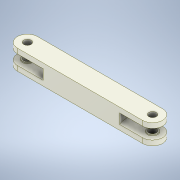
# Autodesk Inventor part: LinkB
Saved by Autodesk Inventor 2022 (Build 260153000, 153)
## iProperties
Created: 2021-11-22
Part Number: LinkB
Material: Plástico ABS
Document SubType Name: Modeling
Designer: JK
Density: 1.06 g/cm^3
Appearance: Suave - Marfil
Author: JK
Autodesk Inventor part; units mm, degrees
ref_plane "YZ Plane" through (0, 0, 0) normal (1, 0, 0) x (0, 1, 0)
ref_plane "XZ Plane" through (0, 0, 0) normal (0, 1, 0) x (-1, 0, 0)
ref_plane "XY Plane" through (0, 0, 0) normal (0, 0, 1) x (1, 0, 0)
sketch "Boceto1" plane through (0, 0, 0) normal (0, 1, 0) x (-1, 0, 0)
  line L0 (-25, 4) -> (25, 4)
  line L1 (25, 4) -> (25, -4)
  line L2 (25, -4) -> (-25, -4)
  line L3 (-25, -4) -> (-25, 4)
  line L4 (-25, 4) -> (25, -4) construction
  line L5 (25, 4) -> (-25, -4) construction
  circle A0 centre (25, 0) radius 4
  circle A1 centre (25, 0) radius 1.5
  circle A2 centre (-25, 0) radius 4
  circle A3 centre (-25, 0) radius 1.5
  point P0 (0, 0)
  point P1 (25, 4)
  point P2 (-25, 4)
  dimension "d0" = 8
  dimension "d1" = 3
  dimension "d2" = 3
  dimension "d15" = 50
  constraints: 12 end point, 4 midpoint, 2 centre point, 2 coincident, 2 horizontal, 2 parallel, 1 perpendicular, 6 other
  measures "d1" diameter of A1
  measures "d2" diameter of A3
  measures "d15" distance of L0.start L0.end
extrude "Extrusión1" add sketch "Boceto1" along normal blind 8 contours A2 L3 A3 | L0 A0 L2 A2 | L3 A3 A2 | A0 L1 A1 | L1 A1 A0
ref_plane "Plano de trabajo1" through (0, 4, 0) normal (0, -1, 0) x (1, 0, 0)
sketch "Boceto2" plane through (0, 4, 0) normal (0, -1, 0) x (1, 0, 0)
  circle A0 centre (25, 0) radius 1.5 projected
  circle A1 centre (25, 0) radius 10
  circle A2 centre (-25, 0) radius 1.5 projected
  circle A3 centre (-25, 0) radius 11
  point P0 (0, 0)
  dimension "d5" = 20
  dimension "d23" = 22
  constraints: 2 centre point, 2 coincident
  measures "d5" diameter of A1
  measures "d23" diameter of A3
extrude "Extrusión2" cut sketch "Boceto2" along normal mid plane 4
sketch "Boceto3" plane through (0, 2, 0) normal (0, 1, 0) x (1, 0, 0)
  circle A0 centre (25, 0) radius 1.5 projected
  circle A1 centre (25, 0) radius 2
  circle A2 centre (-25, 0) radius 1.5 projected
  circle A3 centre (-25, 0) radius 2
  point P0 (0, 0)
  dimension "d9" = 4
  dimension "d24" = 4
  constraints: 2 centre point, 2 coincident
  measures "d9" diameter of A1
  measures "d24" diameter of A3
extrude "Extrusión3" add sketch "Boceto3" along normal up to surface (4 mm away)
sketch "Boceto4" plane through (-25, 0, 4) normal (0, 0, 1) x (1, 0, 0)
  line L0 (40.8348, 5.6) -> (56.0255, 5.6)
  line L1 (56.0255, 5.6) -> (56.0255, 2.4)
  line L2 (56.0255, 2.4) -> (40.8348, 2.4)
  line L3 (40.8348, 2.4) -> (40.8348, 5.6)
  line L4 (40.8348, 5.6) -> (56.0255, 2.4) construction
  line L5 (56.0255, 5.6) -> (40.8348, 2.4) construction
  line L6 (40.8348, 2) -> (40.8348, 6) projected
  line L7 (10.247, 2) -> (10.247, 6) projected
  line L8 (-7.4593, 2.4) -> (10.247, 2.4)
  line L9 (10.247, 2.4) -> (10.247, 5.6)
  line L10 (10.247, 5.6) -> (-7.4593, 5.6)
  line L11 (-7.4593, 5.6) -> (-7.4593, 2.4)
  line L12 (-7.4593, 2.4) -> (10.247, 5.6) construction
  line L13 (10.247, 2.4) -> (-7.4593, 5.6) construction
  point P0 (25, 0)
  point P1 (48.4302, 4)
  point P2 (48.4302, 4)
  point P3 (40.8348, 4)
  point P4 (1.3938, 4)
  dimension "d12" = 3.2
  constraints: 24 end point, 6 midpoint, 4 parallel, 3 collinear, 2 horizontal, 2 perpendicular, 1 horizontal alignment, 1 point on line
  measures "d12" distance between parallel lines of L2 L0
extrude "Extrusión4" cut sketch "Boceto4" against normal through all
sketch "Boceto5" plane through (0, 0, 0) normal (0, -1, 0) x (1, 0, 0)
  circle A0 centre (-25, 0) radius 1.5 projected
  circle A1 centre (-25, 0) radius 8.75
  point P0 (0, 0)
  dimension "d16" = 17.5
  constraints: 1 centre point, 1 coincident
  measures "d16" diameter of A1
sketch "Boceto6" plane through (0, 7.5, 0) normal (0, -1, 0) x (1, 0, 0)
  circle A0 centre (-20, 0) radius 1.5 projected
  circle A1 centre (-20, 0) radius 2
  circle A2 centre (-20, 0) radius 1.5 projected
  point P0 (0, 0)
  dimension "d19" = 4
  constraints: 1 centre point, 1 coincident
  measures "d19" diameter of A1
